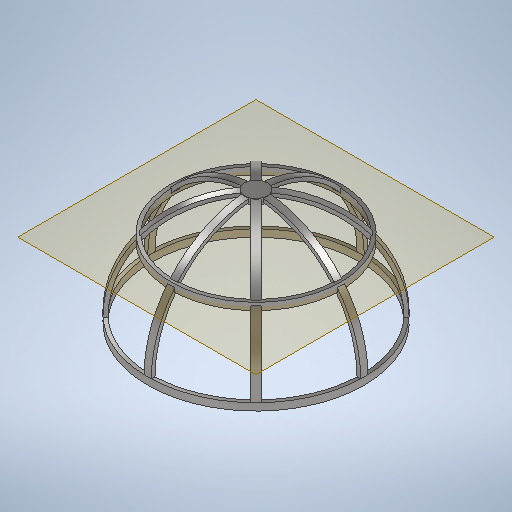
# Autodesk Inventor part: Dome
Saved by Autodesk Inventor 2025.1 (Build 291241000, 241)
## iProperties
Created: 2024-11-07
Part Number: Dome
Material: Steel, Mild
Document SubType Name: Modeling
Designer: smonowar1008
Density: 7.85 g/cm^3
Appearance: Semi-Polished
Author: smonowar1008
Autodesk Inventor part; units mm, degrees
sketch "Sketch1" plane through (0, 0, 0) normal (0, 1, 0) x (-1, 0, 0)
  circle A0 centre (0, 0) radius 95
  circle A1 centre (0, 0) radius 91.825
  dimension "d0" = 190
  dimension "d1" = 183.65
  constraints: 2 centre point, 2 coincident
  measures "d0" diameter of A0
  measures "d1" diameter of A1
extrude "Extrusion1" add sketch "Sketch1" along normal blind 6.35
sketch "Sketch2" plane through (0, 0, 0) normal (1, 0, 0) x (0, 1, 0)
  line L0 (6.35, -95) -> (6.35, 95) projected
  arc A0 (101.35, 0) -> (6.35, 95) centre (6.35, 0) ccw
  arc A1 (98.175, 0) -> (6.35, 91.825) centre (6.35, 0) ccw
  line L1 (101.35, 0) -> (98.175, 0)
  line L2 (6.35, 95) -> (6.35, 91.825)
  point P0 (0, 0)
  dimension "d11" = 91.825
  constraints: 4 end point, 4 point on circle, 2 centre point, 1 coincident, 1 collinear, 1 horizontal, 1 midpoint, 1 point on line
  measures "d11" radius of A1
extrude "Curved Bar 1" add sketch "Sketch2" along normal mid plane 6.35
sketch "Sketch4" plane through (0, 0, 0) normal (1, 0, 0) x (0, 1, 0)
  line L0 (6.35, -95) -> (6.35, 95) projected
  arc A0 (6.35, -95) -> (101.35, 0) centre (6.35, 0) ccw
  arc A1 (6.35, -91.825) -> (98.175, 0) centre (6.35, 0) ccw
  line L1 (101.35, 0) -> (98.175, 0)
  line L2 (6.35, -95) -> (6.35, -91.825)
  point P0 (0, 0)
  point P1 (6.35, 94.946929)
  dimension "d18" = 91.825
  constraints: 4 end point, 4 point on circle, 2 centre point, 1 coincident, 1 horizontal, 1 midpoint, 1 perpendicular
  measures "d18" radius of A1
extrude "Extrusion4" add sketch "Sketch4" along normal mid plane 6.35
sketch "Sketch5" plane through (0, 0, 0) normal (0, 0, 1) x (1, 0, 0)
  line L0 (0, 6.35) -> (-3.175, 6.35) projected
  line L1 (-3.175, 101.35) -> (3.175, 101.35) projected
  line L2 (-3.175, 6.35) -> (-95, 6.35) projected
  arc A0 (0, 101.35) -> (-95, 6.35) centre (0, 6.35) ccw
  arc A1 (0, 98.175) -> (-91.825, 6.35) centre (0, 6.35) ccw
  line L3 (0, 101.35) -> (0, 98.175)
  line L4 (-91.825, 6.35) -> (-95, 6.35)
  point P0 (0, 0)
  point P1 (-91.825, 6.35)
  dimension "d21" = 91.825
  constraints: 4 end point, 4 point on circle, 2 centre point, 1 coincident, 1 midpoint, 1 perpendicular, 1 vertical
  measures "d21" radius of A1
extrude "Extrusion5" add sketch "Sketch5" along normal mid plane 6.35
sketch "Sketch6" plane through (0, 0, 0) normal (0, 0, 1) x (1, 0, 0)
  line L0 (0, 6.35) -> (-3.175, 6.35)
  line L1 (95, 6.35) -> (3.175, 6.35)
  line L2 (0, 101.296929) -> (0, 101.35)
  arc A0 (95, 6.35) -> (0, 101.35) centre (0, 6.35) ccw
  line L3 (0, 6.35) -> (91.825, 6.35)
  arc A1 (91.825, 6.35) -> (0, 98.175) centre (0, 6.35) ccw
  line L4 (95, 6.35) -> (91.825, 6.35)
  line L5 (0, 101.35) -> (0, 98.175)
  point P0 (0, 0)
  dimension "d24" = 91.825
  constraints: 5 point on circle, 4 end point, 2 centre point, 1 coincident, 1 horizontal, 1 perpendicular, 1 point on line
  measures "d24" radius of A1
extrude "Extrusion6" add sketch "Sketch6" along normal mid plane 6.35
ref_plane "Work Plane2" through (0, 0, 0) normal (0.7071068, 0, -0.7071068) x (0, 1, 0)
sketch "Sketch9" plane through (0, 0, 0) normal (0.7071068, 0, -0.7071068) x (0, 1, 0)
  line L0 (6.35, 64.93008) -> (6.35, -64.93008)
  line L1 (0, 95) -> (6.35, 95)
  arc A0 (101.35, 0) -> (6.35, 95) centre (6.35, 0) ccw
  arc A1 (98.175, 0) -> (6.35, 91.825) centre (6.35, 0) ccw
  line L2 (101.35, 0) -> (98.175, 0)
  line L3 (6.35, 95) -> (6.35, 91.825)
  point P0 (0, 0)
  dimension "d35" = 91.825
  constraints: 4 end point, 4 point on circle, 2 centre point, 1 coincident, 1 horizontal, 1 midpoint, 1 perpendicular, 1 point on line
  measures "d35" radius of A1
extrude "Extrusion9" add sketch "Sketch9" along normal mid plane 6.35
sketch "Sketch10" plane through (0, 0, 0) normal (0.7071068, 0, -0.7071068) x (0, 1, 0)
  line L0 (6.35, -64.892553) -> (6.35, 64.892553)
  line L1 (6.35, -95) -> (6.35, -69.382682)
  arc A0 (6.35, -95) -> (101.35, 0) centre (6.35, 0) ccw
  line L2 (6.35, 0) -> (101.35, 0) construction
  line L3 (6.35, 0) -> (6.35, -95) construction
  arc A1 (6.35, -91.825) -> (98.175, 0) centre (6.35, 0) ccw
  line L4 (101.296929, 0) -> (101.323468, 0)
  line L5 (101.35, 0) -> (98.175, 0)
  line L6 (6.35, -95) -> (6.35, -91.825)
  point P0 (0, 0)
  dimension "d38" = 95
  dimension "d39" = 90
  dimension "d40" = 91.825
  constraints: 8 end point, 4 point on circle, 2 centre point, 2 point on line, 1 coincident, 1 midpoint
  measures "d38" radius of A0
  measures "d39" angle of L3 L2
  measures "d40" radius of A1
extrude "Extrusion10" add sketch "Sketch10" along normal mid plane 6.35
ref_plane "Work Plane8" through (-67.175144, 6.35, 67.175144) normal (-0.7071068, 0, -0.7071068) x (0, -1, 0)
sketch "Sketch14" plane through (-67.175144, 6.35, 67.175144) normal (-0.7071068, 0, -0.7071068) x (0, -1, 0)
  line L0 (0, -95) -> (0, -30.06992)
  line L1 (0, 0) -> (0, -25.617318)
  arc A0 (0, 0) -> (-95, -95) centre (0, -95) ccw
  ellipse E0 centre (0, -95) end of major axis (-91.825, -95) minor radius 38.03516 (-91.504516, -91.825) -> (-91.825, -95) ccw
  arc A1 (0, -3.175) -> (-91.825, -95) centre (0, -95) ccw
  line L2 (-95, -95) -> (-91.825, -95)
  line L3 (0, -3.175) -> (0, 0)
  ellipse E1 centre (0, -97.245064) end of major axis (91.825, -97.245064) minor radius 64.93008 (-91.770093, -99.490128) -> (0, -162.175144) ccw
  arc A2 (-95, -95) -> (0, -190) centre (0, -95) ccw
  line L4 (0, -186.825) -> (0, -159.93008)
  arc A3 (-91.825, -95) -> (0, -186.825) centre (0, -95) ccw
  line L5 (-91.825, -95) -> (-95, -95)
  line L6 (0, -190) -> (0, -186.825)
  point P0 (6.35, -95)
  dimension "d51" = 91.825
  dimension "d52" = 91.825
  constraints: 14 end point, 8 point on circle, 4 centre point, 3 coincident, 3 point on line, 8 other
  measures "d51" radius of A1
  measures "d52" radius of A3
extrude "Extrusion13" add sketch "Sketch14" along normal mid plane 6.35 contours L1 A1 L2 A0
extrude "Extrusion14" add sketch "Sketch14" along normal mid plane 6.35 contours L2 A3 L6 A2
ref_plane "Work Plane9" through (0, 101.35, 0) normal (0, 1, 0) x (-1, 0, 0)
sketch "Sketch15" plane through (0, 101.35, 0) normal (0, 1, 0) x (-1, 0, 0)
  circle A0 centre (0, 0) radius 10
  dimension "d57" = 20
  constraints: 1 centre point, 1 coincident
  measures "d57" diameter of A0
extrude "Extrusion15" add sketch "Sketch15" against normal blind 5.08
ref_plane "Work Plane11" through (0, 65, 0) normal (0, 1, 0) x (-1, 0, 0)
sketch "Sketch17" plane through (0, 65, 0) normal (0, 1, 0) x (-1, 0, 0)
  circle A0 centre (0, 0) radius 74.5
  circle A1 centre (0, 0) radius 71.325
  dimension "d66" = 149
  dimension "d67" = 142.65
  constraints: 2 centre point, 2 coincident
  measures "d66" diameter of A0
  measures "d67" diameter of A1
extrude "Extrusion17" add sketch "Sketch17" along normal mid plane 6.35
body "Solid1"
